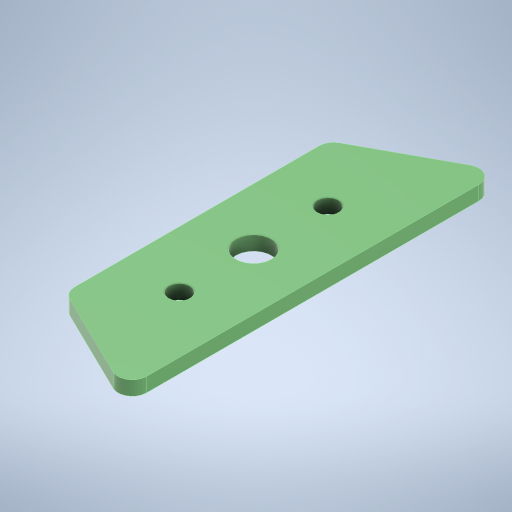
# Autodesk Inventor part: Bumper_Lock_Plate
Saved by Autodesk Inventor 2023 (Build 270158000, 158)
## iProperties
Created: 2023-11-09
Part Number: Bumper_Lock_Plate
Material: Generic
Document SubType Name: Modeling
Designer: adamarnold
Density: 1 g/cm^3
Appearance: Smooth - Dark Forest Green
Author: adamarnold
Autodesk Inventor part; units mm, degrees
ref_plane "YZ Plane" through (0, 0, 0) normal (1, 0, 0) x (0, 1, 0)
ref_plane "XZ Plane" through (0, 0, 0) normal (0, 1, 0) x (-1, 0, 0)
ref_plane "XY Plane" through (0, 0, 0) normal (0, 0, 1) x (1, 0, 0)
sketch "Sketch1" plane through (0, 0, 0) normal (0, 1, 0) x (-1, 0, 0)
  circle A0 centre (0, 0) radius 3.9688
  circle A1 centre (0, -16.6624) radius 2.3813
  circle A2 centre (0, 16.6624) radius 2.3813
  line L0 (12.7, 27.4344) -> (12.7, -27.4344)
  line L1 (-12.7, 36.738) -> (-12.7, -37.8116)
  line L2 (10.9183, 30.2873) -> (-8.1317, 39.591)
  line L3 (12.7, 29.4172) -> (45.9346, 29.4172) construction
  line L4 (-12.7, -0.6673) -> (-17.3723, -0.6673) construction
  line L5 (11.0438, -30.2225) -> (-8.0062, -40.5997)
  arc A3 (-8.1317, 39.591) -> (-12.7, 36.738) centre (-9.525, 36.738) ccw
  arc A4 (12.7, 27.4344) -> (10.9183, 30.2873) centre (9.525, 27.4344) ccw
  arc A5 (11.0438, -30.2225) -> (12.7, -27.4344) centre (9.525, -27.4344) ccw
  arc A6 (-12.7, -37.8116) -> (-8.0062, -40.5997) centre (-9.525, -37.8116) ccw
  point P0 (12.7, -29.3203)
  point P1 (12.7, 0)
  point P2 (-12.7, -43.1566)
  point P3 (-12.7, 41.822)
  dimension "d0" = 7.9375
  dimension "d1" = 4.7625
  dimension "d2" = 16.6624
  dimension "d3" = 4.7625
  dimension "d4" = 16.6624
  dimension "d5" = 12.7
  dimension "d6" = 58.7375
  dimension "d7" = 25.4
  dimension "d8" = 153.97
  dimension "d9" = 3.175
  constraints: 12 end point, 9 point on line, 8 point on circle, 8 tangent, 7 centre point, 3 equal radius, 2 horizontal, 2 vertical alignment, 1 coincident, 1 horizontal alignment, 1 midpoint, 1 parallel, 1 symmetric about line, 1 vertical
  measures "d0" diameter of A0
  measures "d1" diameter of A1
  measures "d2" distance of A1.centre point (0, 0)
  measures "d3" diameter of A2
  measures "d4" distance of point (0, 0) A2.centre
  measures "d5" distance from line of L0 point (0, 0)
  measures "d6" distance of L3.start point (12.7, -29.32)
  measures "d7" distance between parallel lines of L0 L1
  measures "d8" angle of L3 L2
  measures "d9" radius of A3
extrude "Extrusion1" add sketch "Sketch1" along normal blind 3.175
body "Solid1"
